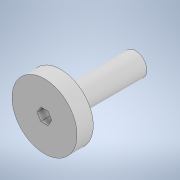
# Autodesk Inventor part: knobForSideGear
Saved by Autodesk Inventor 2022.2 (Build 262287010, 287A)
## iProperties
Created: 2022-09-12
Part Number: knobForSideGear
Material: Generic
Document SubType Name: Modeling
Designer: robst
Density: 1 g/cm^3
Appearance: Default
Author: robst
Autodesk Inventor part; units mm, degrees
ref_plane "YZ Plane" through (0, 0, 0) normal (1, 0, 0) x (0, 1, 0)
ref_plane "XZ Plane" through (0, 0, 0) normal (0, 1, 0) x (-1, 0, 0)
ref_plane "XY Plane" through (0, 0, 0) normal (0, 0, 1) x (1, 0, 0)
sketch "Sketch1" plane through (0, 0, 0) normal (0, 0, 1) x (1, 0, 0)
  line L0 (2.823, 4.8895) -> (5.6459, 0)
  line L1 (5.6459, 0) -> (2.823, -4.8895)
  line L2 (2.823, -4.8895) -> (-2.823, -4.8895)
  line L3 (-2.823, -4.8895) -> (-5.6459, 0)
  line L4 (-5.6459, 0) -> (-2.823, 4.8895)
  line L5 (-2.823, 4.8895) -> (2.823, 4.8895)
  circle A0 centre (0, 0) radius 8.89
  dimension "d0" = 9.779
  dimension "d1" = 17.78
  constraints: 12 end point, 2 coincident, 1 centre point, 1 horizontal, 13 other
  measures "d0" distance between parallel lines of L2 L5
  measures "d1" diameter of A0
extrude "Extrusion1" add sketch "Sketch1" against normal blind 58.42
sketch "Sketch2" plane through (0, 0, 0) normal (0, 0, 1) x (1, 0, 0)
  line L0 (5.6459, 0) -> (2.823, 4.8895) projected
  line L1 (2.823, 4.8895) -> (5.6459, 0)
  line L2 (5.6459, 0) -> (2.823, -4.8895)
  line L3 (2.823, -4.8895) -> (-2.823, -4.8895)
  line L4 (-2.823, -4.8895) -> (-5.6459, 0)
  line L5 (-5.6459, 0) -> (-2.823, 4.8895)
  line L6 (-2.823, 4.8895) -> (2.823, 4.8895)
  circle A0 centre (0, 0) radius 25.4
  point P0 (0, 0)
  point P1 (0, 0)
  dimension "d4" = 50.8
  constraints: 12 end point, 1 centre point, 1 coincident, 13 other
  measures "d4" diameter of A0
extrude "Extrusion2" add sketch "Sketch2" along normal blind 12.7
body "Solid1"
